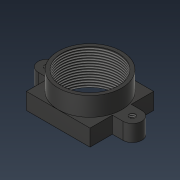
# Autodesk Inventor part: Linsenhalter M12
Saved by Autodesk Inventor 2022.1 (Build 261234020, 234B)
## iProperties
Part Number: Linsenhalter M12
Material: PC/ABS-Kunststoff
Document SubType Name: Modeling
Designer: rYan
Mass: 0.164199 g
Surface Area: 9.11878 cm^2
Volume: 0.459589 cm^3
Density: 0.357273 g/cm^3
Appearance: Glatt - weiß(1)
Author: rYan
Autodesk Inventor part; units mm, degrees
ref_plane "YZ Plane" through (0, 0, 0) normal (1, 0, 0) x (0, 1, 0)
ref_plane "XZ Plane" through (0, 0, 0) normal (0, 1, 0) x (-1, 0, 0)
ref_plane "XY Plane" through (0, 0, 0) normal (0, 0, 1) x (1, 0, 0)
sketch "Skizze1" plane through (0, 0, 0) normal (0, 0, 1) x (1, 0, 0)
  line L0 (-6.75, -6.75) -> (6.75, -6.75)
  line L1 (6.75, 6.75) -> (-6.75, 6.75)
  line L2 (-6.75, -6.75) -> (6.75, 6.75) construction
  line L3 (6.75, -6.75) -> (-6.75, 6.75) construction
  line L4 (-6.75, 2) -> (-9, 2)
  line L5 (-9, -2) -> (-6.75, -2)
  line L6 (6.75, 2) -> (9, 2)
  line L7 (9, -2) -> (6.75, -2)
  arc A0 (-9, 2) -> (-9, -2) centre (-9, 0) ccw
  arc A1 (9, -2) -> (9, 2) centre (9, 0) ccw
  line L8 (-6.75, 6.75) -> (-6.75, 2)
  line L9 (-6.75, -2) -> (-6.75, -6.75)
  line L10 (6.75, -6.75) -> (6.75, -2)
  line L11 (6.75, 2) -> (6.75, 6.75)
  line L12 (0, 9.45) -> (0, -9.45) projected
  line L13 (-15.4, 0) -> (15.4, 0) projected
  point P0 (0, 0)
  dimension "d0" = 13.5
  dimension "d1" = 13.5
  dimension "d2" = 18
  dimension "d3" = 4
  constraints: 24 end point, 7 parallel, 4 point on circle, 4 tangent, 3 horizontal, 3 point on line, 2 centre point, 2 midpoint, 2 perpendicular, 5 other
  measures "d0" distance of L1.start L1.end
  measures "d1" distance between parallel lines of L0 L1
  measures "d2" distance of A1.centre A0.centre
  measures "d3" distance between parallel lines of L7 L6
extrude "Extrusion1" add sketch "Skizze1" along normal blind 3.5
sketch "Skizze4" plane through (0, 0, 3.5) normal (0, 0, 1) x (1, 0, 0)
  arc A0 (-9, 2) -> (-9, -2) centre (-9, 0) ccw projected
  arc A1 (9, -2) -> (9, 2) centre (9, 0) ccw projected
  point P0 (0, 0)
  constraints: 2 coincident
hole "Bohrung1" at (-9, 0, 3.5) at (9, 0, 3.5) direction (0, 0, -1) diameter 1.321 end through all thread size "M1.7x0.35" class "6H" standard "ISO Metric profile"
sketch "Skizze2" plane through (0, 0, 3.5) normal (0, 0, 1) x (1, 0, 0)
  circle A0 centre (0, 0) radius 6.75
  circle A1 centre (0, 0) radius 6
  dimension "d6" = 13.5
  dimension "d7" = 12
  constraints: 2 centre point, 2 coincident
  measures "d6" diameter of A0
  measures "d7" diameter of A1
extrude "Extrusion2" add sketch "Skizze2" along normal blind 4
thread "Gewinde1" size "M12x0.5" class "6H" standard "ANSI Metric M Profile" full length
sketch "Skizze3" plane through (0, 0, 3.5) normal (0, 0, 1) x (1, 0, 0)
  circle A0 centre (0, 0) radius 6 projected
extrude "Extrusion3" cut sketch "Skizze3" against normal through all
